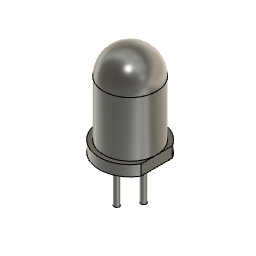
LED_2.54mmp_D5mm (Autodesk Fusion 360 design; units mm, degrees)
Autodesk Fusion 360 part; units mm, degrees
sketch "スケッチ1" plane through (0, 0, 0) normal (0, 0, 1) x (1, 0, 0)
  circle A0 centre (0, 0) radius 2.9
  line L0 (2.5, 1.4697) -> (2.5, -1.4697)
  circle A1 centre (-1.27, 0) radius 0.25
  line L1 (-3.5255, 0) -> (3.8644, 0) construction
  line L2 (0, 3.5138) -> (0, -4.0944) construction
  circle A2 centre (1.27, 0) radius 0.25
  dimension "d1" = 5.8
  dimension "d8" = 2.5
  dimension "d11" = 0.5
  dimension "d14" = 1.27
  constraint coincident A0.centre origin
  constraint vertical L0
  constraint coincident A0 L0.end
  constraint coincident A0 L0.start
  constraint horizontal L1
  constraint coincident A0.centre L1
  constraint coincident A1.centre L1
  constraint vertical L2
  constraint coincident A0.centre L2
  constraint symmetric A1 L2 A2
  measures "d1" diameter of A0
  measures "d8" distance of A0.centre L0
  measures "d11" diameter of A1
  measures "d14" distance of A0.centre A1.centre
extrude "押し出し1" add sketch "スケッチ1" along normal blind 1 contours A0 L0 | A0 L0 | A1 | A2
sketch "スケッチ2" plane through (0, 0, 1) normal (0, 0, 1) x (-1, 0, 0)
  circle A0 centre (0, 0) radius 2.9
  circle A1 centre (0, 0) radius 2.5
  dimension "d4" = 5
  constraint coincident A0.centre A1.centre
  measures "d4" diameter of A1
extrude "押し出し2" add sketch "スケッチ2" along normal blind 7.7 contours A1
fillet "フィレット1" radius 2.5 1 edges at (2.3308, 0.904, 8.7)
extrude "押し出し3" cut sketch "スケッチ1" along normal blind 1 contours A0 L0 picked at (2.5576, -0.3752)
extrude "押し出し4" add sketch "スケッチ1" against normal blind 5 contours A1
extrude "押し出し5" add sketch "スケッチ1" against normal blind 3.5 contours A2
